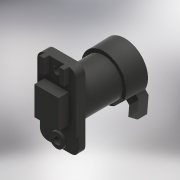
# Autodesk Inventor part: xtion_projector
Saved by Autodesk Inventor 2017 (Build 210142000, 142)
## iProperties
Created: 2016-11-18
Part Number: xtion_projector
Material: Thermoplastic Resin
Document SubType Name: Modeling
Designer: Ali
Density: 1.28 g/cm^3
Appearance: Smooth - Black
Author: Ali
Autodesk Inventor part; units mm, degrees
ref_plane "YZ Plane" through (0, 0, 0) normal (1, 0, 0) x (0, 1, 0)
ref_plane "XZ Plane" through (0, 0, 0) normal (0, 1, 0) x (-1, 0, 0)
sketch "Sketch1" plane through (0, 0, 0) normal (0, 1, 0) x (-1, 0, 0)
  line L0 (-5.3, -10.5) -> (5.3, -10.5)
  line L1 (5.3, -10.5) -> (5.3, 10.5)
  line L2 (5.3, 10.5) -> (-5.3, 10.5)
  line L3 (-5.3, 10.5) -> (-5.3, -10.5)
  line L4 (-5.3, -10.5) -> (5.3, 10.5) construction
  line L5 (5.3, -10.5) -> (-5.3, 10.5) construction
  point P0 (0, 0)
  dimension "d0" = 10.6
  dimension "d1" = 21
  constraints: 12 end point, 2 midpoint, 2 parallel, 1 horizontal, 1 perpendicular
  measures "d0" distance of L2.end L1.end
  measures "d1" distance of L1.end L0.end
extrude "Extrusion1" add sketch "Sketch1" along normal blind 1.8
sketch "Sketch2" plane through (0, 0, 0) normal (0, -1, 0) x (1, 0, 0)
  line L0 (5.3, -10.5) -> (-5.3, -10.5) projected
  line L1 (5.3, 10.5) -> (5.3, -10.5) projected
  line L2 (-5.3, 10.5) -> (5.3, 10.5) projected
  line L3 (-5.3, -10.5) -> (-5.3, 10.5) projected
  line L4 (5.3, 10.5) -> (5.3, -10.5) projected
  line L5 (5.3, -5.4) -> (-5.3, -5.4)
  line L6 (-5.3, -10.5) -> (-5.3, 10.5) projected
  point P0 (0, 0)
  dimension "d4" = 15.9
  constraints: 2 end point, 2 point on line, 1 perpendicular
  measures "d4" distance between parallel lines of L5 L2
extrude "Extrusion2" add sketch "Sketch2" along normal blind 0.7 contours L5 L3 L2 L1
sketch "Sketch3" plane through (0, -0.7, 0) normal (0, -1, 0) x (1, 0, 0)
  line L0 (5.3, 10.5) -> (-5.3, 10.5) projected
  line L1 (-5.3, 10.5) -> (-5.3, -5.4) projected
  line L2 (-5.3, -5.4) -> (5.3, -5.4) projected
  line L3 (5.3, -5.4) -> (5.3, 10.5) projected
  line L4 (-5.3, 10.5) -> (5.3, 10.5) projected
  line L5 (3.35, 10.5) -> (2.1, 10.5)
  line L6 (2.1, 10.5) -> (2.1, 6.5)
  line L7 (2.1, 6.5) -> (3.35, 6.5)
  line L8 (3.35, 6.5) -> (3.35, 10.5)
  line L9 (-2.1, 10.5) -> (-3.35, 10.5)
  line L10 (-3.35, 10.5) -> (-3.35, 6.5)
  line L11 (-3.35, 6.5) -> (-2.1, 6.5)
  line L12 (-2.1, 6.5) -> (-2.1, 10.5)
  line L13 (2.1, 7.4366) -> (-2.1, 7.4366) construction
  line L14 (0, 0) -> (0, 2.1174)
  point P0 (0, 7.4366)
  dimension "d7" = 1.25
  dimension "d8" = 4
  dimension "d9" = 1.25
  dimension "d10" = 4
  dimension "d11" = 4.2
  constraints: 20 end point, 5 point on line, 4 parallel, 3 perpendicular, 2 horizontal, 1 midpoint, 1 vertical
  measures "d7" distance of L7.end L6.end
  measures "d8" distance of L6.end L5.end
  measures "d9" distance of L11.end L10.end
  measures "d10" distance of L10.end L9.end
  measures "d11" distance between parallel lines of L12 L6
extrude "Extrusion3" add sketch "Sketch3" along normal blind 1.4 contours L8 L7 L6 L0 | L12 L11 L10 L0
sketch "Sketch4" plane through (0, -0.7, 0) normal (0, -1, 0) x (1, 0, 0)
  line L0 (3.3, 4.5) -> (-3.3, 4.5)
  line L1 (-3.3, 4.5) -> (-3.3, -3.3)
  line L2 (-3.3, -3.3) -> (3.3, -3.3)
  line L3 (3.3, -3.3) -> (3.3, 4.5)
  line L4 (0, 0) -> (0, 1.0845)
  line L5 (2.1, 10.5) -> (-2.1, 10.5) projected
  point P0 (0, 4.5)
  dimension "d14" = 6.6
  dimension "d15" = 7.8
  dimension "d16" = 6
  constraints: 10 end point, 2 parallel, 1 horizontal, 1 midpoint, 1 perpendicular, 1 point on line, 1 vertical
  measures "d14" distance of L2.end L1.end
  measures "d15" distance of L1.end L0.end
  measures "d16" distance between parallel lines of L0 L5
extrude "Extrusion4" add sketch "Sketch4" along normal blind 2.8
sketch "Sketch5" plane through (0, 0, 0) normal (0, -1, 0) x (1, 0, 0)
  circle A0 centre (0, -8.55) radius 1.95
  line L0 (5.3, -10.5) -> (-5.3, -10.5) projected
  point P0 (0, 0)
  dimension "d19" = 3.9
  constraints: 1 centre point, 1 tangent
  measures "d19" diameter of A0
extrude "Extrusion5" add sketch "Sketch5" along normal up to surface (0.7 mm away)
sketch "Sketch6" plane through (0, -0.7, 0) normal (0, -1, 0) x (1, 0, 0)
  line L0 (3.3, 4.5) -> (3.3, -3.3) projected
  line L1 (3.3, -3.3) -> (-3.3, -3.3) projected
  line L2 (-3.3, -3.3) -> (-3.3, 4.5) projected
  line L3 (-3.3, 4.5) -> (3.3, 4.5) projected
  line L4 (-3.35, 6.5) -> (-3.35, 10.5) projected
  line L5 (-3.35, 10.5) -> (-5.3, 10.5) projected
  line L6 (-5.3, 10.5) -> (-5.3, -5.4) projected
  line L7 (-5.3, -5.4) -> (5.3, -5.4) projected
  line L8 (5.3, -5.4) -> (5.3, 10.5) projected
  line L9 (5.3, 10.5) -> (3.35, 10.5) projected
  line L10 (3.35, 10.5) -> (3.35, 6.5) projected
  line L11 (3.35, 6.5) -> (2.1, 6.5) projected
  line L12 (2.1, 6.5) -> (2.1, 10.5) projected
  line L13 (2.1, 10.5) -> (-2.1, 10.5) projected
  line L14 (-2.1, 10.5) -> (-2.1, 6.5) projected
  line L15 (-2.1, 6.5) -> (-3.35, 6.5) projected
  circle A0 centre (0, -8.55) radius 1.95 projected
  point P0 (0, 0)
  point P1 (0, 7.95)
  dimension "d22" = 16.5
  constraints: 1 coincident
  measures "d22" distance of point (0, 7.95) point (0, -8.55)
hole "Hole1" at (0, -0.7, 7.95) at (0, -0.7, -8.55) direction (0, 1, 0) diameter 2 end through all
fillet "Fillet1" radius 2.1 4 edges at (-5.3, 0.55, 10.5) (5.3, 0.55, 10.5) (5.3, 0.9, -10.5) (-5.3, 0.9, -10.5)
sketch "Sketch7" plane through (0, 1.8, 0) normal (0, 1, 0) x (1, 0, 0)
  circle A0 centre (0, 0) radius 5.175
  dimension "d31" = 10.35
  constraints: 1 centre point, 1 coincident
  measures "d31" diameter of A0
extrude "Extrusion6" add sketch "Sketch7" along normal blind 10.3
sketch "Sketch8" plane through (0, 0, 0) normal (1, 0, 0) x (0, 1, 0)
  line L0 (12.1, -5.175) -> (12.1, 5.175) projected
  line L1 (1.8, 5.175) -> (1.8, -5.175) projected
  line L2 (12.1, -5.175) -> (12.1, 5.175) projected
  line L3 (12.1, -5.175) -> (12.1, -6.15)
  line L4 (12.1, -6.15) -> (17.8961, -6.29)
  line L5 (17.8961, -6.29) -> (17.8961, -5.79)
  line L6 (17.8961, 0) -> (12.1, 0)
  line L7 (17.8961, -5.79) -> (13.2961, -3.5781)
  line L8 (13.2961, -3.5781) -> (13.2961, 0)
  point P0 (0, 0)
  dimension "d34" = 12.3
  dimension "d35" = 12.58
  dimension "d37" = 2.6
  dimension "d38" = 4.6
  dimension "d39" = 0.5
  constraints: 12 end point, 1 midpoint, 1 parallel, 1 perpendicular, 1 point on line, 1 vertical
  measures "d34" diameter of L3.end L6
  measures "d35" diameter of L4.end L6
  measures "d37" distance from line of L4 L7.end
  measures "d38" distance from line of L7.end L5
  measures "d39" distance of L4.end L5.end
revolve "Revolution1" add sketch "Sketch8" angle 360 about axis through (0, 17.8961, 0) along (0, -1, 0)
chamfer "Chamfer1" distance 0.12 angle 45 1 edges at (-5.175, 1.8, 0)
sketch "Sketch9" plane through (0, 17.8961, 0) normal (0, 1, 0) x (1, 0, 0)
  line L0 (0, 0) -> (4.9828, 4.9828) construction
  line L1 (0, 0) -> (0, 2.6372) construction
  dimension "d43" = 45
  constraints: 4 end point, 1 coincident, 1 vertical
  measures "d43" angle of L0 L1
ref_plane "Work Plane2" through (4.4477, 17.8961, -4.4477) normal (-0.7071, 0, 0.7071) x (0, -1, 0)
sketch "Sketch11" plane through (4.4477, 17.8961, -4.4477) normal (-0.7071, 0, 0.7071) x (0, -1, 0)
  line L0 (0, -6.29) -> (0, 6.29) projected
  line L1 (5.7961, -6.15) -> (5.7961, 6.15) projected
  line L2 (5.7961, 5.175) -> (5.7961, -5.175) projected
  line L3 (5.7961, 1.825) -> (2.6, 1.825)
  line L4 (2.6, 1.825) -> (2.6, -1.825)
  line L5 (2.6, -1.825) -> (5.7961, -1.825)
  line L6 (5.7961, -1.825) -> (5.7961, 1.825)
  line L7 (0, 0) -> (0.8817, 0)
  point P0 (17.8961, 0)
  point P1 (2.6, 0)
  dimension "d45" = 3.65
  dimension "d46" = 2.6
  constraints: 10 end point, 2 horizontal, 2 midpoint, 2 parallel, 2 point on line, 1 perpendicular
  measures "d45" distance between parallel lines of L5 L3
  measures "d46" distance between parallel lines of L0 L4
extrude "Extrusion7" cut sketch "Sketch11" along normal blind 3.3
sketch "Sketch12" plane through (4.4477, 17.8961, -4.4477) normal (-0.7071, 0, 0.7071) x (0, -1, 0)
  line L0 (5.7961, 1.825) -> (2.6, 1.825) projected
  line L1 (2.6, 1.825) -> (2.6, -1.825) projected
  line L2 (2.6, -1.825) -> (5.7961, -1.825) projected
  line L3 (5.7961, 1.825) -> (5.7961, -1.825) projected
  line L4 (0, -6.29) -> (0, 6.29) projected
  line L5 (0, -6.29) -> (0, 6.29) projected
  line L6 (2.6, 1.825) -> (0, 1.825)
  line L7 (0, 1.825) -> (0, -1.825)
  line L8 (0, -1.825) -> (2.6, -1.825)
  line L9 (2.6, -1.825) -> (2.6, 1.825)
  point P0 (17.8961, 0)
  constraints: 8 end point, 2 parallel, 1 horizontal, 1 perpendicular, 1 point on line
extrude "Extrusion8" add sketch "Sketch12" along normal blind 0.3 and the other way blind 1 contours L1 L8 L4 L6
sketch "Sketch13" plane through (6.4453, 15.2961, -3.8643) normal (0.7071, 0, 0.7071) x (0.7071, 0, -0.7071)
  line L0 (-1.3, 0) -> (-1.3, 1.4344) projected
  line L1 (-1.3, 0) -> (0, 0) projected
  line L2 (0, 2.6) -> (0, 0) projected
  line L3 (0, 2.6) -> (-1.2706, 2.6) projected
  line L4 (0, 2.6) -> (-1.2706, 2.6) projected
  line L5 (0, 2.6) -> (3.0642, 0.0288)
  line L6 (3.0642, 0.0288) -> (1.7143, -1.5798)
  line L7 (1.7143, -1.5798) -> (-0.1685, 0)
  line L8 (-1.3, 0) -> (0, 0) projected
  point P0 (-7.29, -15.2961)
  dimension "d53" = 2.6
  dimension "d54" = 2.1
  dimension "d55" = 40
  dimension "d56" = 4
  constraints: 6 end point, 1 parallel, 1 perpendicular, 1 point on line, 1 other
  measures "d53" distance between parallel lines of L1 L3
  measures "d54" distance between parallel lines of L7 L5
  measures "d55" angle of L5 L3
  measures "d56" distance of L2.start L5.end
extrude "Extrusion9" add sketch "Sketch13" against normal up to surface (3.65 mm away)
body "Solid1"
